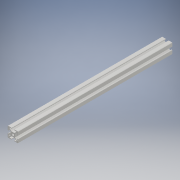
# Autodesk Inventor part: 2020 Extrusion 250mm
Saved by Autodesk Inventor 2018 (Build 220112000, 112)
## iProperties
Created: 2018-05-10
Part Number: 2020 Extrusion 250mm
Material: Aluminum 6061
Document SubType Name: Modeling
Designer: Hans Rueckschnat
Density: 2.7 g/cm^3
Appearance: Aluminum - Flat
Author: Hans Rueckschnat
Autodesk Inventor part; units mm, degrees
ref_plane "YZ Plane" through (0, 0, 0) normal (1, 0, 0) x (0, 1, 0)
ref_plane "XZ Plane" through (0, 0, 0) normal (0, 1, 0) x (-1, 0, 0)
ref_plane "XY Plane" through (0, 0, 0) normal (0, 0, 1) x (1, 0, 0)
sketch "Sketch1" plane through (0, 0, 0) normal (0, 1, 0) x (-1, 0, 0)
  line L0 (-2.9393, 4) -> (2.9393, 4)
  line L1 (4, 2.9393) -> (4, -2.9393)
  line L2 (2.9393, -4) -> (-2.9393, -4)
  line L3 (-4, -2.9393) -> (-4, 2.9393)
  circle A0 centre (0, 0) radius 2.15
  line L4 (-2.9393, 4) -> (-6.75, 7.8107)
  line L5 (-7.8107, 6.75) -> (-4, 2.9393)
  line L6 (4, -2.9393) -> (7.8107, -6.75)
  line L7 (-10, 10) -> (-2.5, 10)
  line L8 (2.5, 10) -> (10, 10)
  line L9 (10, -10) -> (2.5, -10)
  line L10 (-2.5, -10) -> (-10, -10)
  line L11 (10, 10) -> (10, 2.5)
  line L12 (10, -2.5) -> (10, -10)
  line L13 (-10, -10) -> (-10, -2.5)
  line L14 (-10, 2.5) -> (-10, 10)
  line L15 (-8.5, 2.5) -> (-8.5, 6.75)
  line L16 (-6.75, 8.5) -> (-2.5, 8.5)
  line L17 (2.5, 10) -> (2.5, 8.5)
  line L18 (10, 2.5) -> (8.5, 2.5)
  line L19 (10, -2.5) -> (8.5, -2.5)
  line L20 (2.5, -8.5) -> (2.5, -10)
  line L21 (-2.5, -8.5) -> (-2.5, -10)
  line L22 (-8.5, -2.5) -> (-10, -2.5)
  line L23 (-8.5, 2.5) -> (-10, 2.5)
  line L24 (-2.5, 10) -> (-2.5, 8.5)
  line L25 (-7.8107, 6.75) -> (-8.5, 6.75)
  line L26 (-6.75, 8.5) -> (-6.75, 7.8107)
  line L27 (6.75, 8.5) -> (6.75, 7.8107)
  line L28 (8.5, 6.75) -> (7.8107, 6.75)
  line L29 (8.5, 6.75) -> (8.5, 2.5)
  line L30 (2.5, 8.5) -> (6.75, 8.5)
  line L31 (6.75, 7.8107) -> (2.9393, 4)
  line L32 (7.8107, 6.75) -> (4, 2.9393)
  line L33 (2.9393, -4) -> (6.75, -7.8107)
  line L34 (8.5, -2.5) -> (8.5, -6.75)
  line L35 (6.75, -8.5) -> (2.5, -8.5)
  line L36 (8.5, -6.75) -> (7.8107, -6.75)
  line L37 (6.75, -7.8107) -> (6.75, -8.5)
  line L38 (-2.5, -8.5) -> (-6.75, -8.5)
  line L39 (-2.9393, -4) -> (-6.75, -7.8107)
  line L40 (-8.5, -6.75) -> (-8.5, -2.5)
  line L41 (-4, -2.9393) -> (-7.8107, -6.75)
  line L42 (-6.75, -7.8107) -> (-6.75, -8.5)
  line L43 (-7.8107, -6.75) -> (-8.5, -6.75)
  dimension "d0" = 20
  dimension "d1" = 20
  dimension "d26" = 1.5
  dimension "d27" = 1.5
  dimension "d32" = 7.5
  dimension "d33" = 5
  dimension "d34" = 7.5
  dimension "d35" = 7.5
  dimension "d40" = 6
  dimension "d41" = 13.5
  constraints: 88 end point, 19 parallel, 9 horizontal, 7 perpendicular, 7 vertical, 1 centre point
  measures "d0" distance of L9.start L10.end
  measures "d1" distance of L8.end L9.start
  measures "d26" distance between parallel lines of L14 L15
  measures "d27" distance between parallel lines of L7 L16
  measures "d32" distance between parallel lines of L9 L19
  measures "d33" distance between parallel lines of L19 L18
  measures "d34" distance between parallel lines of L18 L8
  measures "d35" distance of L8.start L8.end
  measures "d40" distance between parallel lines of L14 L3
  measures "d41" distance between parallel lines of L42 L37
extrude "Extrusion1" add sketch "Sketch1" along normal blind 300
chamfer "Chamfer1" distance 0.5 angle 45 12 edges at (-10, 150, 2.5) (-10, 150, -2.5) (-2.5, 150, 10) (2.5, 150, 10) (10, 150, 2.5) (10, 150, -2.5) (2.5, 150, -10) (-2.5, 150, -10) (-10, 150, 10) (-10, 150, -10) (10, 150, -10) (10, 150, 10)
body "Solid1"
